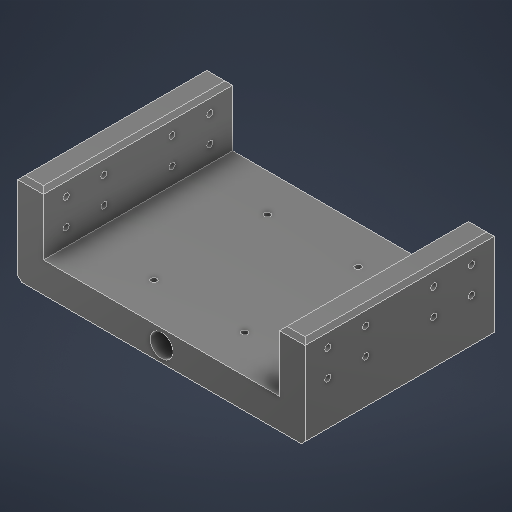
# Autodesk Inventor part: SACMI DPA TILES GRIP FIXED SUPPORT
Saved by Autodesk Inventor 2025 (Build 290162000, 162)
## iProperties
Created: 2024-05-27
Part Number: SACMI DPA TILES GRIP FIXED SUPPORT
Material: Generic
Document SubType Name: Modeling
Designer: zulet
Density: 1 g/cm^3
Appearance: Smooth - Black
Author: zulet
Autodesk Inventor part; units mm, degrees
ref_plane "YZ Plane" through (0, 0, 0) normal (1, 0, 0) x (0, 1, 0)
ref_plane "XZ Plane" through (0, 0, 0) normal (0, 1, 0) x (-1, 0, 0)
ref_plane "XY Plane" through (0, 0, 0) normal (0, 0, 1) x (1, 0, 0)
sketch "Sketch1" plane through (0, 0, 0) normal (0, 1, 0) x (-1, 0, 0)
  line L0 (190, -125) -> (-190, -125)
  line L1 (-190, -125) -> (-190, 125)
  line L2 (-190, 125) -> (190, 125)
  line L3 (190, 125) -> (190, -125)
  line L4 (190, -125) -> (-190, 125) construction
  line L5 (-190, -125) -> (190, 125) construction
  line L6 (-60, 75) -> (60, 75) construction
  line L7 (60, 75) -> (60, -75) construction
  line L8 (60, -75) -> (-60, -75) construction
  line L9 (-60, -75) -> (-60, 75) construction
  line L10 (-60, 75) -> (60, -75) construction
  line L11 (60, 75) -> (-60, -75) construction
  line L12 (-156, 125) -> (156, 125)
  line L13 (156, 125) -> (156, -125)
  line L14 (156, -125) -> (-156, -125)
  line L15 (-156, -125) -> (-156, 125)
  line L16 (-156, 125) -> (156, -125) construction
  line L17 (156, 125) -> (-156, -125) construction
  point P0 (0, 0)
  dimension "d0" = 380
  dimension "d1" = 250
  dimension "d2" = 120
  dimension "d3" = 150
  dimension "d16" = 312
  constraints: 36 end point, 6 midpoint, 6 parallel, 4 coincident, 3 horizontal, 3 perpendicular, 1 point on line
  measures "d0" distance of L1.end L2.end
  measures "d1" distance of L0.end L1.end
  measures "d2" distance of L7.end L8.end
  measures "d3" distance of L6.end L7.end
  measures "d16" distance of L13.end L14.end
extrude "Extrusion1" add sketch "Sketch1" along normal blind 40
hole "Hole1" at (-60, 0, -75) at (60, 0, -75) at (60, 0, 75) at (-60, 0, 75) direction (0, 1, 0) diameter 8 end through all
sketch "Sketch2" plane through (-190, 0, 125) normal (0, 0, 1) x (1, 0, 0)
  line L0 (0, 0) -> (380, 0) construction
  line L1 (0, 40) -> (380, 40) construction
  line L2 (380, 0) -> (0, 40) construction
  line L3 (0, 0) -> (380, 40) construction
  circle A0 centre (190, 20) radius 15
  point P0 (190, 0)
  dimension "d13" = 30
  constraints: 4 end point, 1 centre point, 1 midpoint
  measures "d13" diameter of A0
extrude "Extrusion2" cut sketch "Sketch2" against normal through all
extrude "Extrusion3" add sketch "Sketch1" along normal blind 120 contours L0 L13 L2 L3 | L0 L1 L2 L15
sketch "Sketch3" plane through (-190, 0, -125) normal (-1, 0, 0) x (0, 0, 1)
  line L0 (170, 97.5) -> (220, 97.5) construction
  line L1 (220, 97.5) -> (220, 62.5) construction
  line L2 (220, 62.5) -> (170, 62.5) construction
  line L3 (170, 62.5) -> (170, 97.5) construction
  line L4 (170, 97.5) -> (220, 62.5) construction
  line L5 (220, 97.5) -> (170, 62.5) construction
  line L6 (0, 0) -> (250, 0) construction
  line L7 (125, 0) -> (125, 120) construction
  line L8 (0, 120) -> (250, 120) construction
  line L9 (80, 97.5) -> (30, 97.5) construction
  line L10 (30, 97.5) -> (30, 62.5) construction
  line L11 (30, 62.5) -> (80, 62.5) construction
  line L12 (80, 62.5) -> (80, 97.5) construction
  line L13 (80, 97.5) -> (30, 62.5) construction
  line L14 (30, 97.5) -> (80, 62.5) construction
  point P0 (195, 80)
  point P1 (55, 80)
  dimension "d19" = 50
  dimension "d20" = 35
  dimension "d21" = 62.5
  dimension "d22" = 70
  constraints: 26 end point, 9 symmetric about line, 8 coincident, 3 midpoint, 2 parallel, 1 horizontal, 1 perpendicular
  measures "d19" distance of L1.end L2.end
  measures "d20" distance of L0.end L1.end
  measures "d21" distance between parallel lines of L6 L2
  measures "d22" distance from line of L7 point (195, 80)
hole "Hole2" at (-190, 97.5, 45) at (-190, 97.5, 95) at (-190, 62.5, 95) at (-190, 62.5, 45) at (-190, 62.5, -45) at (-190, 62.5, -95) at (-190, 97.5, -95) at (-190, 97.5, -45) direction (1, 0, 0) diameter 8 end through all
chamfer "Chamfer1" distance 5 angle 45 10 edges at (-190, 120, 0) (-173, 120, 125) (-156, 120, 0) (-173, 120, -125) (156, 120, 0) (190, 120, 0) (173, 120, -125) (173, 120, 125) (-190, 0, 0) (190, 0, 0)
body "Solid1"
